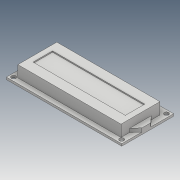
# Autodesk Inventor part: 1806LCD
Saved by Autodesk Inventor 2018 (Build 220112000, 112)
## iProperties
Created: 2018-10-30
Part Number: 1806LCD
Material: 일반
Document SubType Name: Modeling
Designer: dhksr
Density: 1 g/cm^3
Appearance: 기본값
Author: dhksr
Autodesk Inventor part; units mm, degrees
ref_plane "YZ Plane" through (0, 0, 0) normal (1, 0, 0) x (0, 1, 0)
ref_plane "XZ Plane" through (0, 0, 0) normal (0, 1, 0) x (-1, 0, 0)
ref_plane "XY Plane" through (0, 0, 0) normal (0, 0, 1) x (1, 0, 0)
sketch "스케치1" plane through (0, 0, 0) normal (0, 0, 1) x (1, 0, 0)
  line L0 (0, 0) -> (80, 0)
  line L1 (80, 0) -> (80, 36)
  line L2 (80, 36) -> (0, 36)
  line L3 (0, 36) -> (0, 0)
  dimension "d0" = 80
  dimension "d1" = 36
  constraints: 8 end point, 2 parallel, 1 horizontal, 1 perpendicular
  measures "d0" distance of L2.end L1.end
  measures "d1" distance of L1.end L0.end
extrude "돌출1" add sketch "스케치1" along normal blind 1.5
sketch "스케치2" plane through (0, 0, 1.5) normal (0, 0, 1) x (1, 0, 0)
  line L0 (80, 36) -> (0, 36) projected
  line L1 (0, 36) -> (0, 0) projected
  line L2 (4.5, 30.5) -> (76, 30.5)
  line L3 (76, 30.5) -> (76, 3.5)
  line L4 (76, 3.5) -> (4.5, 3.5)
  line L5 (4.5, 3.5) -> (4.5, 30.5)
  dimension "d4" = 71.5
  dimension "d5" = 27
  dimension "d6" = 5.5
  dimension "d7" = 4.5
  constraints: 8 end point, 2 parallel, 1 horizontal, 1 perpendicular
  measures "d4" distance of L3.end L4.end
  measures "d5" distance of L2.end L3.end
  measures "d6" distance between parallel lines of L0 L2
  measures "d7" distance between parallel lines of L1 L5
extrude "돌출2" add sketch "스케치2" along normal blind 8
sketch "스케치3" plane through (0, 0, 1.5) normal (0, 0, 1) x (1, 0, 0)
  line L0 (76, 30.5) -> (76, 3.5) projected
  line L1 (76, 24.5) -> (76, 9.5)
  line L2 (80, 20) -> (80, 14)
  line L3 (76, 24.5) -> (80, 20)
  line L4 (80, 14) -> (76, 9.5)
  point P0 (80, 36)
  point P1 (76, 17)
  point P2 (80, 17)
  point P3 (76, 17)
  dimension "d10" = 15
  dimension "d11" = 6
  constraints: 8 end point, 3 midpoint, 2 vertical, 2 vertical alignment, 1 coincident, 1 horizontal alignment
  measures "d10" distance of L1.start L1.end
  measures "d11" distance of L2.start L2.end
extrude "돌출3" add sketch "스케치3" along normal blind 2.5
sketch "스케치5" plane through (0, 0, 9.5) normal (0, 0, 1) x (1, 0, 0)
  line L0 (76, 30.5) -> (4.5, 30.5) projected
  line L1 (4.5, 30.5) -> (4.5, 3.5) projected
  line L2 (72.25, 23.75) -> (8.25, 23.75)
  line L3 (8.25, 23.75) -> (8.25, 10.25)
  line L4 (8.25, 10.25) -> (72.25, 10.25)
  line L5 (72.25, 10.25) -> (72.25, 23.75)
  line L6 (72.25, 23.75) -> (8.25, 10.25) construction
  line L7 (8.25, 23.75) -> (72.25, 10.25) construction
  point P0 (0, 0)
  point P1 (40.25, 17)
  point P2 (40.25, 17)
  point P3 (4.5, 17)
  point P4 (40.25, 17)
  point P5 (40.25, 30.5)
  dimension "d15" = 64
  dimension "d16" = 13.5
  constraints: 12 end point, 6 midpoint, 2 parallel, 1 horizontal, 1 horizontal alignment, 1 perpendicular, 1 vertical alignment
  measures "d15" distance of L4.end L3.end
  measures "d16" distance of L2.end L3.end
extrude "돌출4" cut sketch "스케치5" against normal blind 0.8
sketch "스케치6" plane through (0, 0, 1.5) normal (0, 0, 1) x (1, 0, 0)
  line L0 (80, 20) -> (80, 36) projected
  line L1 (80, 36) -> (0, 36) projected
  line L2 (0, 36) -> (0, 0) projected
  line L3 (0, 0) -> (80, 0) projected
  circle A0 centre (2.5, 33.5) radius 1.5
  circle A1 centre (77.5, 33.5) radius 1.5
  circle A2 centre (77.5, 2.5) radius 1.5
  circle A3 centre (2.5, 2.5) radius 1.5
  dimension "d19" = 80
  dimension "d20" = 3
  dimension "d21" = 3
  dimension "d22" = 3
  dimension "d23" = 3
  dimension "d24" = 1
  dimension "d25" = 1
  dimension "d26" = 1
  dimension "d27" = 1
  constraints: 4 centre point, 2 horizontal alignment, 2 vertical alignment
  measures "d19" distance between parallel lines of L0 L2
  measures "d20" diameter of A0
  measures "d21" diameter of A1
  measures "d22" diameter of A2
  measures "d23" diameter of A3
  measures "d24" distance edge to line of A1 L0
  measures "d25" distance edge to line of A1 L1
  measures "d26" distance edge to line of A0 L2
  measures "d27" distance edge to line of A3 L3
extrude "돌출5" cut sketch "스케치6" against normal through all
sketch "스케치7" plane through (0, 0, 9.5) normal (0, 0, 1) x (1, 0, 0)
  line L0 (8.25, 10.25) -> (8.25, 23.75) projected
  line L1 (8.25, 23.75) -> (72.25, 23.75) projected
  line L2 (72.25, 23.75) -> (72.25, 10.25) projected
  line L3 (72.25, 10.25) -> (8.25, 10.25) projected
  line L4 (76, 30.5) -> (4.5, 30.5) projected
  line L5 (4.5, 30.5) -> (4.5, 3.5) projected
  line L6 (4.5, 3.5) -> (76, 3.5) projected
  line L7 (76, 3.5) -> (76, 30.5) projected
  circle A0 centre (77.5, 2.5) radius 1.5 projected
  circle A1 centre (2.5, 33.5) radius 1.5 projected
  circle A2 centre (77.5, 33.5) radius 1.5 projected
  circle A3 centre (2.5, 2.5) radius 1.5 projected
  line L8 (76, 24.5) -> (80, 20) projected
  line L9 (80, 20) -> (80, 36) projected
  line L10 (80, 36) -> (0, 36) projected
  line L11 (0, 36) -> (0, 0) projected
  line L12 (0, 0) -> (80, 0) projected
  line L13 (80, 0) -> (80, 14) projected
  line L14 (80, 14) -> (76, 9.5) projected
  line L15 (76, 9.5) -> (76, 3.5) projected
  line L16 (76, 3.5) -> (4.5, 3.5) projected
  line L17 (4.5, 3.5) -> (4.5, 30.5) projected
  line L18 (4.5, 30.5) -> (76, 30.5) projected
  line L19 (76, 30.5) -> (76, 24.5) projected
  line L20 (2.5, 33.5) -> (77.5, 33.5)
  line L21 (77.5, 33.5) -> (77.5, 2.5)
  line L22 (77.5, 2.5) -> (2.5, 2.5)
  line L23 (2.5, 2.5) -> (2.5, 33.5)
  line L24 (40, 33.5) -> (40, -15.5556)
  line L25 (2.5, 18) -> (93.9243, 18)
  line L26 (8.25, 17) -> (83.8017, 17) construction
  line L27 (40.25, 23.75) -> (40.25, -12.7239) construction
  line L28 (40, 18) -> (40.25, 18)
  line L29 (40.25, 18) -> (40.25, 17)
  dimension "d30" = 80
  dimension "d31" = 36
  dimension "d32" = 75
  dimension "d33" = 31
  dimension "d34" = 71.5
  dimension "d35" = 27
  dimension "d36" = 1
  dimension "d37" = 0.25
  constraints: 20 end point, 6 point on line, 4 midpoint, 3 horizontal, 3 parallel, 1 perpendicular, 1 vertical
  measures "d30" distance of L9.end L10.end
  measures "d31" distance of L10.end L11.end
  measures "d32" distance of L20.start L20.end
  measures "d33" distance of L22.end L20.start
  measures "d34" distance of L4.start L4.end
  measures "d35" distance of L4.end L5.end
  measures "d36" distance of L29.end L28.end
  measures "d37" distance of L28.end L28.start
